Autodesk Inventor part; units mm, degrees
(part 2 of 2)
  line L178 (74.8347, 20.9788) -> (74.8347, 19.1865)
  spline S274 degree 2 poles (74.8347, 19.1865) (74.8347, 19.0015) (74.6588, 19.0015) knots 0 0 0 1 1 1
  spline S275 degree 2 poles (74.6588, 19.0015) (74.4799, 19.0015) (74.4799, 19.1865) knots 0 0 0 1 1 1
  line L179 (74.4799, 19.1865) -> (74.4799, 22.9894)
  line L180 (74.4799, 22.9894) -> (76.0023, 22.9894)
  spline S276 degree 2 poles (76.0023, 22.9894) (76.5118, 22.9894) (76.7726, 22.6983) knots 0 0 0 1 1 1
  spline S277 degree 2 poles (76.7726, 22.6983) (77.0121, 22.4314) (77.0121, 21.9613) knots 0 0 0 1 1 1
  spline S278 degree 2 poles (76.6573, 21.9613) (76.6573, 22.6285) (76.0023, 22.6285) knots 0 0 0 1 1 1
  line L181 (76.0023, 22.6285) -> (74.8347, 22.6285)
  line L182 (74.8347, 22.6285) -> (74.8347, 21.3457)
  line L183 (74.8347, 21.3457) -> (76.0993, 21.3457)
  spline S279 degree 2 poles (76.0993, 21.3457) (76.3662, 21.3457) (76.6573, 21.6823) (76.6573, 21.9613) knots 0 0 0 1 2 2 2
  line L184 (80.1327, 19.0531) -> (77.7005, 19.0531)
  line L185 (77.7005, 19.0531) -> (77.7005, 22.8044)
  spline S280 degree 2 poles (77.7005, 22.8044) (77.7005, 22.9894) (77.8795, 22.9894) knots 0 0 0 1 1 1
  spline S281 degree 2 poles (77.8795, 22.9894) (78.0553, 22.9894) (78.0553, 22.8044) knots 0 0 0 1 1 1
  line L186 (78.0553, 22.8044) -> (78.0553, 19.4139)
  line L187 (78.0553, 19.4139) -> (80.1327, 19.4139)
  spline S282 degree 2 poles (80.1327, 19.4139) (80.3116, 19.4139) (80.3116, 19.235) knots 0 0 0 1 1 1
  spline S283 degree 2 poles (80.3116, 19.235) (80.3116, 19.0531) (80.1327, 19.0531) knots 0 0 0 1 1 1
  spline S284 degree 2 poles (83.702, 21.1425) (83.702, 20.069) (83.138, 19.511) knots 0 0 0 1 1 1
  spline S285 degree 2 poles (83.138, 19.511) (82.674, 19.0591) (82.0129, 19.0591) knots 0 0 0 1 1 1
  line L188 (82.0129, 19.0591) -> (80.997, 19.0591)
  line L189 (80.997, 19.0591) -> (80.997, 22.9894)
  line L190 (80.997, 22.9894) -> (82.0068, 22.9894)
  spline S286 degree 2 poles (82.0068, 22.9894) (82.6619, 22.9894) (83.138, 22.5588) knots 0 0 0 1 1 1
  spline S287 degree 2 poles (83.138, 22.5588) (83.702, 22.0493) (83.702, 21.1425) knots 0 0 0 1 1 1
  spline S288 degree 2 poles (83.3472, 21.1456) (83.3472, 21.8643) (82.9014, 22.2767) knots 0 0 0 1 1 1
  spline S289 degree 2 poles (82.9014, 22.2767) (82.5224, 22.6194) (82.0068, 22.6194) knots 0 0 0 1 1 1
  line L191 (82.0068, 22.6194) -> (81.3518, 22.6194)
  line L192 (81.3518, 22.6194) -> (81.3518, 19.42)
  line L193 (81.3518, 19.42) -> (82.0129, 19.42)
  spline S290 degree 2 poles (82.0129, 19.42) (82.5406, 19.42) (82.9075, 19.8021) knots 0 0 0 1 1 1
  spline S291 degree 2 poles (82.9075, 19.8021) (83.3472, 20.2631) (83.3472, 21.1456) knots 0 0 0 1 1 1
  point P0 (43.75, 0)
  point P1 (20.5, 42)
  point P2 (20.5, 21)
  dimension "d71" = 10
  dimension "d72" = 65
  dimension "d73" = 2
  constraints: 3 collinear, 2 horizontal alignment, 2 midpoint, 2 vertical, 4 other
  measures "d71" distance of L0.end L1.end
  measures "d72" distance of L0.start L0.end
  measures "d73" distance between parallel lines of L9 L1
emboss "Emboss1" sketch "Sketch9" operation cut depth 1 direction (0, 0, -1)
body "Solid1"
